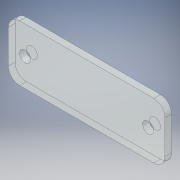
# Autodesk Inventor part: new connect acr
Saved by Autodesk Inventor 2019 (Build 230136000, 136)
## iProperties
Created: 2020-03-01
Part Number: new connect acr
Material: Glass
Document SubType Name: Modeling
Designer: KiranM
Density: 2.18 g/cm^3
Appearance: Clear
Author: KiranM
Autodesk Inventor part; units mm, degrees
ref_plane "YZ Plane" through (0, 0, 0) normal (1, 0, 0) x (0, 1, 0)
ref_plane "XZ Plane" through (0, 0, 0) normal (0, 1, 0) x (-1, 0, 0)
ref_plane "XY Plane" through (0, 0, 0) normal (0, 0, 1) x (1, 0, 0)
sketch "Sketch1" plane through (0, 0, 0) normal (0, 0, 1) x (1, 0, 0)
  line L0 (0, 0) -> (0, -25)
  line L1 (0, -25) -> (70, -25)
  line L2 (70, -25) -> (70, 0)
  line L3 (70, 0) -> (0, 0)
  dimension "d0" = 25
  dimension "d1" = 70
  constraints: 8 end point, 3 perpendicular, 1 vertical
  measures "d0" distance of L0.start L0.end
  measures "d1" distance of L0.end L1.end
extrude "Extrusion1" add sketch "Sketch1" along normal blind 3
fillet "Fillet1" radius 5 1 edges at (70, 0, 1.5)
fillet "Fillet2" radius 5 1 edges at (70, -25, 1.5)
fillet "Fillet3" radius 5 1 edges at (0, -25, 1.5)
fillet "Fillet4" radius 5 1 edges at (0, 0, 1.5)
sketch "Sketch2" plane through (0, 0, 0) normal (0, 0, -1) x (-1, 0, 0)
  circle A0 centre (-62.4991, -12.5) radius 2.5
  circle A1 centre (-7.5, -12.5) radius 2.5
  point P0 (0, 0)
  constraints: 2 centre point
extrude "Extrusion2" cut sketch "Sketch2" against normal through all
body "Solid1"
